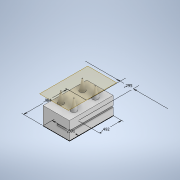
# Autodesk Inventor part: photovoltaic_clip2
Saved by Autodesk Inventor 2020.2 (Build 242310000, 310)
## iProperties
Created: 2020-04-12
Part Number: photovoltaic_clip2
Material: Generic
Document SubType Name: Modeling
Designer: DELL
Density: 1 g/cm^3
Appearance: Default
Author: DELL
## iProperties of the stored document _3DPrint.ipt
Created: 2020-04-12
Part Number: _3DPrint
Material: Generic
Document SubType Name: Modeling
Designer: DELL
Density: 1 g/cm^3
Appearance: Default
Author: DELL
Autodesk Inventor part; units mm, degrees
ref_plane "YZ Plane" through (0, 0, 0) normal (1, 0, 0) x (0, 1, 0)
ref_plane "XZ Plane" through (0, 0, 0) normal (0, 1, 0) x (-1, 0, 0)
ref_plane "XY Plane" through (0, 0, 0) normal (0, 0, 1) x (1, 0, 0)
sketch "Sketch1" plane through (0, 0, 0) normal (0, 1, 0) x (-1, 0, 0)
  line L0 (7.5, 12.5) -> (-7.5, 12.5)
  line L1 (-7.5, 12.5) -> (-7.5, -12.5)
  line L2 (-7.5, -12.5) -> (7.5, -12.5)
  line L3 (7.5, -12.5) -> (7.5, 12.5)
  point P0 (0, 0)
  dimension "d0" = 25
  dimension "d1" = 15
  dimension "d2" = 7.5
  dimension "d3" = 12.5
  constraints: 8 end point, 2 parallel, 1 horizontal, 1 perpendicular
  measures "d0" distance of L2.end L0.start
  measures "d1" distance of L0.start L0.end
  measures "d2" distance from line of L3 point (0, 0)
  measures "d3" distance from line of point (0, 0) L2
extrude "Extrusion1" add sketch "Sketch1" along normal blind 10
sketch "Sketch3" plane through (7.5, 0, 12.5) normal (1, 0, 0) x (0, 0, -1)
  line L0 (0, 0) -> (0, 10) projected
  line L1 (0, 5) -> (25, 5)
  line L2 (25, 5) -> (25, 4.2)
  line L3 (25, 4.2) -> (0, 4.2)
  line L4 (0, 4.2) -> (0, 5)
  point P0 (12.5, 0)
  dimension "d8" = 0.8
  dimension "d9" = 25
  constraints: 8 end point, 2 parallel, 1 horizontal, 1 midpoint, 1 perpendicular
  measures "d8" distance of L2.end L1.end
  measures "d9" distance of L1.start L1.end
extrude "Extrusion2" cut sketch "Sketch3" against normal blind 7
sketch "Sketch4" plane through (0, 10, 0) normal (0, 1, 0) x (1, 0, 0)
  circle A0 centre (3.69, -6.15) radius 1.5316
  line L0 (-7.5, -12.5) -> (7.5, -12.5) projected
  line L1 (7.5, -12.5) -> (7.5, 12.5) projected
  circle A1 centre (-3.69, -6.15) radius 1.5367
  line L2 (-7.5, 12.5) -> (-7.5, -12.5) projected
  point P0 (0, 0)
  dimension "d12" = 6.35
  dimension "d13" = 3.81
  dimension "d14" = 3.0631
  dimension "d15" = 3.81
  dimension "d16" = 3.0734
  dimension "d17" = 6.35
  constraints: 2 centre point
  measures "d12" distance from line of L0 A0.centre
  measures "d13" distance from line of L1 A0.centre
  measures "d14" diameter of A0
  measures "d15" distance from line of L2 A1.centre
  measures "d16" diameter of A1
  measures "d17" distance from line of L0 A1.centre
sketch "Sketch5" plane through (0, 10, 0) normal (0, 1, 0) x (1, 0, 0)
  circle A0 centre (3.69, 6.15) radius 1.5367
  circle A1 centre (-3.69, 6.15) radius 1.5367
  line L0 (7.5, 12.5) -> (-7.5, 12.5) projected
  line L1 (-7.5, 12.5) -> (-7.5, -12.5) projected
  line L2 (7.5, -12.5) -> (7.5, 12.5) projected
  point P0 (0, 0)
  dimension "d18" = 6.35
  dimension "d19" = 6.35
  dimension "d20" = 3.81
  dimension "d21" = 3.81
  dimension "d22" = 3.0734
  dimension "d23" = 3.0734
  constraints: 2 centre point
  measures "d18" distance from line of L0 A0.centre
  measures "d19" distance from line of L0 A1.centre
  measures "d20" distance from line of L1 A1.centre
  measures "d21" distance from line of L2 A0.centre
  measures "d22" diameter of A0
  measures "d23" diameter of A1
ref_plane "Work Plane1" through (0, 16, 0) normal (0, 1, 0) x (1, 0, 0)
sketch "Sketch6" plane through (0, 16, 0) normal (0, 1, 0) x (1, 0, 0)
  circle A0 centre (3.69, 6.15) radius 0.254
  line L0 (7.5, 12.5) -> (-7.5, 12.5) projected
  line L1 (7.5, -12.5) -> (7.5, 12.5) projected
  point P0 (0, 0)
  dimension "d41" = 0.508
  dimension "d42" = 6.35
  dimension "d43" = 3.81
  constraints: 1 centre point
  measures "d41" diameter of A0
  measures "d42" distance from line of L0 A0.centre
  measures "d43" distance from line of L1 A0.centre
loft "Loft1" add profiles "Sketch6", "Sketch5" contours all / A0
sketch "Sketch7" plane through (0, 16, 0) normal (0, 1, 0) x (1, 0, 0)
  circle A0 centre (3.69, -6.15) radius 0.254
  line L0 (7.5, -12.5) -> (7.5, 12.5) projected
  line L1 (-7.5, -12.5) -> (7.5, -12.5) projected
  point P0 (0, 0)
  dimension "d44" = 0.508
  dimension "d45" = 3.81
  dimension "d46" = 6.35
  constraints: 1 centre point
  measures "d44" diameter of A0
  measures "d45" distance from line of L0 A0.centre
  measures "d46" distance from line of L1 A0.centre
loft "Loft2" add profiles "Sketch4", "Sketch7" contours A0 / all
sketch "Sketch10" plane through (0, 16, 0) normal (0, 1, 0) x (1, 0, 0)
  circle A0 centre (-3.69, -6.15) radius 0.254
  line L0 (-7.5, 12.5) -> (-7.5, -12.5) projected
  line L1 (-7.5, -12.5) -> (7.5, -12.5) projected
  point P0 (0, 0)
  dimension "d53" = 3.81
  dimension "d54" = 6.35
  dimension "d55" = 0.508
  constraints: 1 centre point
  measures "d53" distance from line of L0 A0.centre
  measures "d54" distance from line of L1 A0.centre
  measures "d55" diameter of A0
loft "Loft3" add profiles "Sketch4", "Sketch10" contours A1 / all
sketch "Sketch11" plane through (0, 16, 0) normal (0, 1, 0) x (1, 0, 0)
  circle A0 centre (-3.69, 6.15) radius 0.254
  line L0 (-7.5, 12.5) -> (-7.5, -12.5) projected
  line L1 (7.5, 12.5) -> (-7.5, 12.5) projected
  point P0 (0, 0)
  dimension "d60" = 0.508
  dimension "d61" = 3.81
  dimension "d62" = 6.35
  constraints: 1 centre point
  measures "d60" diameter of A0
  measures "d61" distance from line of L0 A0.centre
  measures "d62" distance from line of L1 A0.centre
loft "Loft4" add profiles "Sketch5", "Sketch11" contours A1 / all
body "Solid1"
